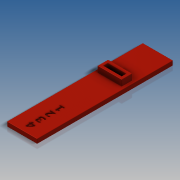
# Autodesk Inventor part: 11237-Red
Saved by Autodesk Inventor 2016 SP2 (Build 200236200, 236)
## iProperties
Created: 2015-08-26
Part Number: 11237-Red
Material: ABS Plastic
Document SubType Name: Modeling
Designer: D. Kohfeld
Density: 1.06 g/cm^3
Appearance: Red
Mass: 0.382311 g
Surface Area: 7.38339 cm^2
Volume: 0.360671 cm^3
Author: D. Kohfeld
Autodesk Inventor part; units mm, degrees
ref_plane "YZ Plane" through (0, 0, 0) normal (1, 0, 0) x (0, 1, 0)
ref_plane "XZ Plane" through (0, 0, 0) normal (0, 1, 0) x (-1, 0, 0)
ref_plane "XY Plane" through (0, 0, 0) normal (0, 0, 1) x (1, 0, 0)
sketch "Sketch2" plane through (0, 0, 0) normal (0, 1, 0) x (-1, 0, 0)
  line L0 (-4, 18) -> (4, 18)
  line L1 (4, 18) -> (4, -18)
  line L2 (4, -18) -> (-4, -18)
  line L3 (-4, -18) -> (-4, 18)
  line L4 (-3.2, -5.2) -> (3.2, -5.2)
  line L5 (3.2, -5.2) -> (3.2, -8)
  line L6 (3.2, -8) -> (-3.2, -8)
  line L7 (-3.2, -8) -> (-3.2, -5.2)
  line L8 (-2.4, -6) -> (2.4, -6)
  line L9 (2.4, -6) -> (2.4, -7.2)
  line L10 (2.4, -7.2) -> (-2.4, -7.2)
  line L11 (-2.4, -7.2) -> (-2.4, -6)
  line L12 (-0.8, -8.4) -> (0.8, -8.4)
  line L13 (0.8, -8.4) -> (0.8, -9.6)
  line L14 (0.8, -9.6) -> (-0.8, -9.6)
  line L15 (-0.8, -9.6) -> (-0.8, -8.4)
  line L16 (-0.92, 16.6) -> (0.92, 16.6) construction
  line L17 (0.92, 16.6) -> (0.92, 14.76) construction
  line L18 (0.92, 14.76) -> (-0.92, 14.76) construction
  line L19 (-0.92, 14.76) -> (-0.92, 16.6) construction
  line L20 (-0.92, 14.08) -> (0.92, 14.08) construction
  line L21 (0.92, 14.08) -> (0.92, 12.24) construction
  line L22 (0.92, 12.24) -> (-0.92, 12.24) construction
  line L23 (-0.92, 12.24) -> (-0.92, 14.08) construction
  line L24 (-0.92, 11.56) -> (0.92, 11.56) construction
  line L25 (0.92, 11.56) -> (0.92, 9.72) construction
  line L26 (0.92, 9.72) -> (-0.92, 9.72) construction
  line L27 (-0.92, 9.72) -> (-0.92, 11.56) construction
  line L28 (-0.92, 9.04) -> (0.92, 9.04) construction
  line L29 (0.92, 9.04) -> (0.92, 7.2) construction
  line L30 (0.92, 7.2) -> (-0.92, 7.2) construction
  line L31 (-0.92, 7.2) -> (-0.92, 9.04) construction
  line L32 (0.92, 14.76) -> (0.92, 14.08) construction
  line L33 (0.92, 12.24) -> (0.92, 11.56) construction
  line L34 (0.92, 9.72) -> (0.92, 9.04) construction
  line L35 (0.7991, 15.1858) -> (0.5482, 15.1858)
  line L36 (0.5482, 15.1858) -> (0.5482, 14.7577)
  line L37 (0.5482, 14.7577) -> (0.0946, 14.7577)
  line L38 (0.0946, 14.7577) -> (0.0946, 15.1858)
  line L39 (0.0946, 15.1858) -> (-0.7961, 15.1858)
  line L40 (-0.7961, 15.1858) -> (-0.7961, 15.5343)
  line L41 (-0.7961, 15.5343) -> (0.0646, 16.6023)
  line L42 (0.0646, 16.6023) -> (0.5482, 16.6023)
  line L43 (0.5482, 16.6023) -> (0.5482, 15.5223)
  line L44 (0.5482, 15.5223) -> (0.7991, 15.5223)
  line L45 (0.7991, 15.5223) -> (0.7991, 15.1858)
  line L46 (0.0946, 15.5223) -> (0.0946, 16.1892)
  line L47 (0.0946, 16.1892) -> (-0.4416, 15.5223)
  line L48 (-0.4416, 15.5223) -> (0.0946, 15.5223)
  spline S0 degree 2 poles (0.5933, 13.1022) (0.6534, 13.0496) (0.7255, 12.9114) (0.7255, 12.7973) knots 0 0 0 1 2 2 2
  spline S1 degree 2 poles (0.7255, 12.7973) (0.7255, 12.6666) (0.6233, 12.4413) (0.5167, 12.3617) knots 0 0 0 1 2 2 2
  spline S2 degree 2 poles (0.5167, 12.3617) (0.4131, 12.2836) (0.1322, 12.2009) (-0.0676, 12.2009) knots 0 0 0 1 2 2 2
  spline S3 degree 2 poles (-0.0676, 12.2009) (-0.2974, 12.2009) (-0.6248, 12.273) (-0.727, 12.3166) knots 0 0 0 1 2 2 2
  line L49 (-0.727, 12.3166) -> (-0.727, 12.7207)
  line L50 (-0.727, 12.7207) -> (-0.6789, 12.7207)
  spline S4 degree 2 poles (-0.6789, 12.7207) (-0.5723, 12.6561) (-0.2764, 12.5629) (-0.1547, 12.5629) knots 0 0 0 1 2 2 2
  spline S5 degree 2 poles (-0.1547, 12.5629) (-0.0826, 12.5629) (0.0856, 12.587) (0.1427, 12.626) knots 0 0 0 1 2 2 2
  spline S6 degree 2 poles (0.1427, 12.626) (0.1893, 12.6576) (0.2433, 12.7447) (0.2433, 12.8273) knots 0 0 0 1 2 2 2
  spline S7 degree 2 poles (0.2433, 12.8273) (0.2433, 12.9084) (0.1697, 12.9955) (0.1081, 13.0136) knots 0 0 0 1 2 2 2
  spline S8 degree 2 poles (0.1081, 13.0136) (0.0481, 13.0346) (-0.1232, 13.0376) (-0.1953, 13.0376) knots 0 0 0 1 2 2 2
  line L51 (-0.1953, 13.0376) -> (-0.2974, 13.0376)
  line L52 (-0.2974, 13.0376) -> (-0.2974, 13.3665)
  line L53 (-0.2974, 13.3665) -> (-0.1923, 13.3665)
  spline S9 degree 2 poles (-0.1923, 13.3665) (-0.0961, 13.3665) (0.0526, 13.3785) (0.1051, 13.4011) knots 0 0 0 1 2 2 2
  spline S10 degree 2 poles (0.1051, 13.4011) (0.1592, 13.4251) (0.2133, 13.5032) (0.2133, 13.5783) knots 0 0 0 1 2 2 2
  spline S11 degree 2 poles (0.2133, 13.5783) (0.2133, 13.6354) (0.1562, 13.703) (0.1127, 13.7225) knots 0 0 0 1 2 2 2
  spline S12 degree 2 poles (0.1127, 13.7225) (0.0646, 13.745) (-0.0661, 13.7601) (-0.1127, 13.7601) knots 0 0 0 1 2 2 2
  spline S13 degree 2 poles (-0.1127, 13.7601) (-0.2298, 13.7601) (-0.5017, 13.679) (-0.6294, 13.6039) knots 0 0 0 1 2 2 2
  line L54 (-0.6294, 13.6039) -> (-0.6744, 13.6039)
  line L55 (-0.6744, 13.6039) -> (-0.6744, 14.0034)
  spline S14 degree 2 poles (-0.6744, 14.0034) (-0.5723, 14.044) (-0.2238, 14.1191) (-0.0451, 14.1191) knots 0 0 0 1 2 2 2
  spline S15 degree 2 poles (-0.0451, 14.1191) (0.1292, 14.1191) (0.392, 14.059) (0.4776, 14.0079) knots 0 0 0 1 2 2 2
  spline S16 degree 2 poles (0.4776, 14.0079) (0.5783, 13.9463) (0.6774, 13.7736) (0.6774, 13.6579) knots 0 0 0 1 2 2 2
  spline S17 degree 2 poles (0.6774, 13.6579) (0.6774, 13.5047) (0.4867, 13.2629) (0.3304, 13.2298) knots 0 0 0 1 2 2 2
  line L56 (0.3304, 13.2298) -> (0.3304, 13.2118)
  spline S18 degree 2 poles (0.3304, 13.2118) (0.3935, 13.2028) (0.5347, 13.1517) (0.5933, 13.1022) knots 0 0 0 1 2 2 2
  line L57 (0.7736, 9.702) -> (-0.6714, 9.702)
  line L58 (-0.6714, 9.702) -> (-0.6714, 10.0054)
  spline S19 degree 2 poles (-0.6714, 10.0054) (-0.5062, 10.1256) (-0.1727, 10.3944) (-0.0736, 10.492) knots 0 0 0 1 2 2 2
  spline S20 degree 2 poles (-0.0736, 10.492) (0.0766, 10.6377) (0.2028, 10.8525) (0.2028, 10.9577) knots 0 0 0 1 2 2 2
  spline S21 degree 2 poles (0.2028, 10.9577) (0.2028, 11.0839) (0.0406, 11.2205) (-0.1112, 11.2205) knots 0 0 0 1 2 2 2
  spline S22 degree 2 poles (-0.1112, 11.2205) (-0.2253, 11.2205) (-0.4761, 11.1274) (-0.5843, 11.0538) knots 0 0 0 1 2 2 2
  line L59 (-0.5843, 11.0538) -> (-0.6233, 11.0538)
  line L60 (-0.6233, 11.0538) -> (-0.6233, 11.4624)
  spline S23 degree 2 poles (-0.6233, 11.4624) (-0.5362, 11.5014) (-0.1938, 11.578) (-0.021, 11.578) knots 0 0 0 1 2 2 2
  spline S24 degree 2 poles (-0.021, 11.578) (0.3244, 11.578) (0.6879, 11.2881) (0.6879, 11.0223) knots 0 0 0 1 2 2 2
  spline S25 degree 2 poles (0.6879, 11.0223) (0.6879, 10.8465) (0.5137, 10.5326) (0.335, 10.3659) knots 0 0 0 1 2 2 2
  spline S26 degree 2 poles (0.335, 10.3659) (0.2223, 10.2622) (-0.006, 10.088) (-0.0541, 10.0535) knots 0 0 0 1 2 2 2
  line L61 (-0.0541, 10.0535) -> (0.7736, 10.0535)
  line L62 (0.7736, 10.0535) -> (0.7736, 9.702)
  line L63 (0.6579, 7.1977) -> (-0.5708, 7.1977)
  line L64 (-0.5708, 7.1977) -> (-0.5708, 7.5192)
  line L65 (-0.5708, 7.5192) -> (-0.1832, 7.5192)
  line L66 (-0.1832, 7.5192) -> (-0.1832, 8.491)
  line L67 (-0.1832, 8.491) -> (-0.5708, 8.491)
  line L68 (-0.5708, 8.491) -> (-0.5708, 8.7914)
  spline S27 degree 2 poles (-0.5708, 8.7914) (-0.4822, 8.7914) (-0.3184, 8.8124) (-0.2644, 8.838) knots 0 0 0 1 2 2 2
  spline S28 degree 2 poles (-0.2644, 8.838) (-0.1998, 8.8695) (-0.1367, 8.9687) (-0.1307, 9.0423) knots 0 0 0 1 2 2 2
  line L69 (-0.1307, 9.0423) -> (0.2779, 9.0423)
  line L70 (0.2779, 9.0423) -> (0.2779, 7.5192)
  line L71 (0.2779, 7.5192) -> (0.6579, 7.5192)
  line L72 (0.6579, 7.5192) -> (0.6579, 7.1977)
  point P0 (0, 0)
  point P1 (0, 18)
  point P2 (-4, 0)
  point P3 (0, -5.2)
  point P4 (0, -6)
  point P5 (-2.4, -6.6)
  point P6 (-3.2, -6.6)
  point P7 (0, -8.4)
  point P8 (0, 14.76)
  point P9 (0, 12.24)
  point P10 (0, 9.72)
  point P11 (0, 7.2)
  dimension "d0" = 8
  dimension "d1" = 36
  dimension "d4" = 6.4
  dimension "d5" = 2.8
  dimension "d6" = 0.8
  dimension "d7" = 0.8
  dimension "d8" = 10
  dimension "d9" = 1.2
  dimension "d10" = 1.6
  dimension "d11" = 0.4
  dimension "d16" = 0.68
  dimension "d18" = 1.84
  dimension "d19" = 1.4
  constraints: 38 end point, 11 midpoint, 8 parallel, 8 vertical alignment, 7 horizontal, 6 equal length, 4 perpendicular, 3 vertical, 2 horizontal alignment, 8 other
  measures "d0" distance of L0.start L0.end
  measures "d1" distance of L0.end L1.end
  measures "d4" distance of L4.start L4.end
  measures "d5" distance of L6.end L4.start
  measures "d6" distance between parallel lines of L7 L11
  measures "d7" distance between parallel lines of L8 L4
  measures "d8" distance between parallel lines of L2 L6
  measures "d9" distance of L14.end L12.start
  measures "d10" distance of L13.end L14.end
  measures "d11" distance between parallel lines of L12 L6
  measures "d16" distance between parallel lines of L26 L28
  measures "d18" distance between parallel lines of L18 L16
  measures "d19" distance from line of L16.end L0
extrude "Extrusion1" add sketch "Sketch2" against normal blind 1.2 contours L0 L1 L2 L3 | L4 L5 L6 L7 | L8 L9 L10 L11 | L12 L13 L14 L15 | L35 L36 L37 L38 L39 L40 L41 L42 L43 L44 L45 | L48 L47 L46 | S0 S1 S2 S3 L49 L50 S4 S5 S6 S7 S8 L51 L52 L53 S9 S10 S11 S12 S13 L54 L55 S14 S15 S16 S17 L56 S18 | L57 L58 S19 S20 S21 S22 L59 L60 S23 S24 S25 S26 L61 L62 | L63 L64 L65 L66 L67 L68 S27 S28 L69 L70 L71 L72
extrude "Extrusion2" add sketch "Sketch2" along normal blind 1.6 contours L4 L5 L6 L7
extrude "Extrusion3" cut sketch "Sketch2" against normal blind 0.8 contours L12 L13 L14 L15
extrude "Extrusion4" cut sketch "Sketch2" against normal blind 0.4 contours L35 L36 L37 L38 L39 L40 L41 L42 L43 L44 L45 | S0 S1 S2 S3 L49 L50 S4 S5 S6 S7 S8 L51 L52 L53 S9 S10 S11 S12 S13 L54 L55 S14 S15 S16 S17 L56 S18 | L57 L58 S19 S20 S21 S22 L59 L60 S23 S24 S25 S26 L61 L62 | L63 L64 L65 L66 L67 L68 S27 S28 L69 L70 L71 L72
fillet "Fillet1" radius 0.1 28 edges at (-4, 0, 0) (-4, -1.2, 0) (-4, -0.6, 18) (0, 0, 18) (0, -1.2, 18) (4, 0, 0) (4, -0.6, 18) (4, -1.2, 0) (3.2, 0.8, -5.2) (3.2, 1.6, -6.6) (0, 1.6, -5.2) (-3.2, 0.8, -5.2) (-3.2, 1.6, -6.6) (0, 1.6, -8) (-3.2, 0.8, -8) (3.2, 0.8, -8) (0, 1.6, -7.2) (2.4, 1.6, -6.6) (0, 1.6, -6) (-2.4, 1.6, -6.6) (-4, -0.6, -18) (0, -1.2, -18) (0, 0, -18) (4, -0.6, -18) (0, 0, -8.4) (-0.8, 0, -9) (0, 0, -9.6) (0.8, 0, -9)
equation "\"d0\" = lu"
equation "\"d7\" = d6"
equation "\"d10\" = wall"
equation "\"d20\" = wall"
equation "\"lu\" = 8"
equation "\"wall\" = 1.6"
body "Solid1"
